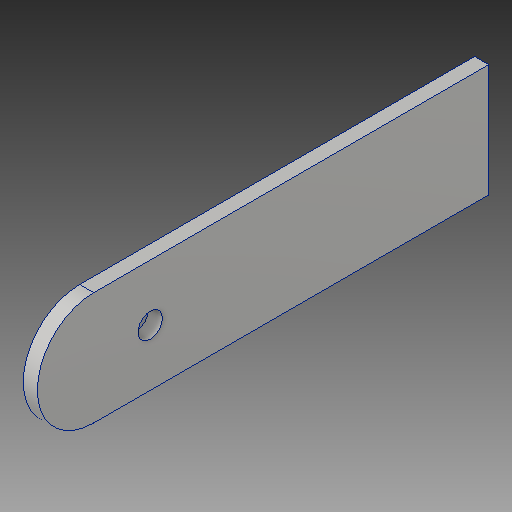
# Autodesk Inventor part: thing4
Saved by Autodesk Inventor 2017 (Build 210142000, 142)
## iProperties
Created: 2018-01-30
Part Number: thing4
Material: Aluminum 6061
Document SubType Name: Modeling
Designer: S346905847
Density: 2.7 g/cm^3
Appearance: Aluminum - Flat
Author: S346905847
Autodesk Inventor part; units mm, degrees
ref_plane "YZ Plane" through (0, 0, 0) normal (1, 0, 0) x (0, 1, 0)
ref_plane "XZ Plane" through (0, 0, 0) normal (0, 1, 0) x (-1, 0, 0)
ref_plane "XY Plane" through (0, 0, 0) normal (0, 0, 1) x (1, 0, 0)
sketch "Sketch1" plane through (0, 0, 0) normal (1, 0, 0) x (0, 1, 0)
  circle A0 centre (0, 0) radius 12.7
  line L0 (0, 12.7) -> (0, -88.9)
  line L1 (12.7, 0) -> (12.7, -88.9)
  line L2 (12.7, -88.9) -> (0, -88.9)
  line L3 (-12.7, -88.9) -> (-12.7, 0)
  line L4 (0, -88.9) -> (-12.7, -88.9)
  dimension "d0" = 25.4
  dimension "d1" = 101.6
  constraints: 10 end point, 3 point on circle, 2 tangent, 2 vertical, 1 centre point, 1 coincident, 1 horizontal, 1 perpendicular, 1 point on line
  measures "d0" diameter of A0
  measures "d1" distance of L0.start L0.end
extrude "Extrusion1" add sketch "Sketch1" along normal blind 3.175
sketch "Sketch6" plane through (3.175, 0, 0) normal (1, 0, 0) x (0, 0, -1)
  circle A0 centre (12.7, 0) radius 2.75
  point P0 (0, 0)
  dimension "d8" = 5.5
  constraints: 1 centre point
  measures "d8" diameter of A0
extrude "Extrusion2" cut sketch "Sketch6" against normal through all
body "Solid1"
